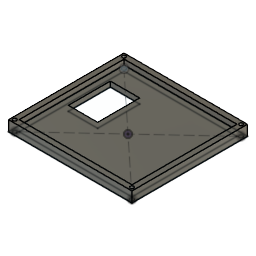
Bottom box road eye (Autodesk Fusion 360 design; units mm, degrees)
Autodesk Fusion 360 part; units mm, degrees
sketch "Sketch1" plane through (0, 0, 0) normal (0, 0, 1) x (1, 0, 0)
  line L0 (53.7502, -49.9897) -> (-53.7502, -49.9897)
  line L1 (-53.7502, -49.9897) -> (-53.7502, 49.9897)
  line L2 (-53.7502, 49.9897) -> (53.7502, 49.9897)
  line L3 (53.7502, 49.9897) -> (53.7502, -49.9897)
  line L4 (53.7502, -49.9897) -> (-53.7502, 49.9897) construction
  line L5 (-53.7502, -49.9897) -> (53.7502, 49.9897) construction
  line L6 (58.826, -55.0656) -> (-58.826, -55.0656)
  line L7 (-58.826, -55.0656) -> (-58.826, 55.0656)
  line L8 (-58.826, 55.0656) -> (58.826, 55.0656)
  line L9 (58.826, 55.0656) -> (58.826, -55.0656)
  circle A0 centre (-55.826, 52.0656) radius 1.7
  circle A1 centre (-55.826, 52.0656) radius 1.7
  circle A2 centre (55.826, 52.0656) radius 1.7
  circle A3 centre (55.826, -52.0656) radius 1.7
  circle A4 centre (-55.826, -52.0656) radius 1.7
  line L10 (-47.1513, 30.2997) -> (-19.2113, 30.2997)
  line L11 (-19.2113, 30.2997) -> (-19.2113, -9.7053)
  line L12 (-19.2113, -9.7053) -> (-47.1513, -9.7053)
  line L13 (-47.1513, -9.7053) -> (-47.1513, 30.2997)
  dimension "d1" = 107.5004
  dimension "d2" = 99.9795
  dimension "d3" = -5.0758
  dimension "d4" = 3.4
  dimension "d5" = 3
  dimension "d6" = 3
  dimension "d7" = 3.4
  dimension "d8" = 3.4
  dimension "d9" = 3
  dimension "d10" = 3
  dimension "d11" = 3.4
  dimension "d12" = 3
  dimension "d13" = 3
  dimension "d14" = 3.4
  dimension "d15" = 3
  dimension "d16" = 3
  dimension "d17" = 6.5989
  dimension "d18" = 19.6901
  dimension "d19" = 27.94
  dimension "d20" = 40.005
  constraint horizontal L0
  constraint perpendicular L0 L1
  constraint parallel L0 L2
  constraint parallel L1 L3
  constraint coincident L4 origin
  constraint coincident L5 origin
  constraint perpendicular L1 L10
  constraint perpendicular L10 L11
  constraint perpendicular L1 L12
  constraint perpendicular L10 L13
  measures "d1" distance of L1.end L2.end
  measures "d2" distance of L0.end L1.end
  measures "d4" diameter of A0
  measures "d5" distance of L7 A0.centre
  measures "d6" distance of L8 A0.centre
  measures "d7" diameter of A1
  measures "d8" diameter of A2
  measures "d9" distance of L8 A2.centre
  measures "d10" distance of L9 A2.centre
  measures "d11" diameter of A3
  measures "d12" distance of L6 A3.centre
  measures "d13" distance of L9 A3.centre
  measures "d14" diameter of A4
  measures "d15" distance of L7 A4.centre
  measures "d16" distance of L6 A4.centre
  measures "d17" distance of L1 L10.start
  measures "d18" distance of L2 L10
  measures "d19" distance of L10.start L10.end
  measures "d20" distance of L10.start L12.end
extrude "Extrude1" add sketch "Sketch1" along normal blind 5 contours L0 L1 L2 L3
extrude "Extrude2" add sketch "Sketch1" along normal blind 10 contours L6 L7 L8 L9
extrude "Extrude3" add sketch "Sketch1" along normal blind 5 contours A0 A1 | A2 | A3 | A4
